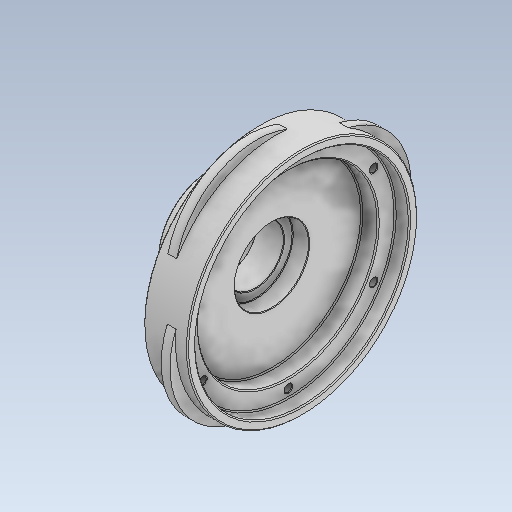
# Autodesk Inventor part: Peça21
Saved by Autodesk Inventor 2021 (Build 250183000, 183)
## iProperties
Category: 41
Created: 2021-07-19
Part Number: Peça21
Material: Genérico
Document SubType Name: Modeling
Designer: Giovanni
Density: 1 g/cm^3
Appearance: Padrão
User Status: 1:6
Author: Giovanni
Keywords: 27
Autodesk Inventor part; units mm, degrees
ref_plane "YZ Plane" through (0, 0, 0) normal (1, 0, 0) x (0, 1, 0)
sketch "Esboço1" plane through (0, 0, 0) normal (0, 0, 1) x (1, 0, 0)
  line L0 (0, 0) -> (100, 0)
  line L1 (0, 0) -> (0, 47.5)
  line L2 (0, 47.5) -> (35, 47.5)
  line L3 (35, 47.5) -> (35, 90)
  line L4 (35, 90) -> (45, 90)
  line L5 (45, 90) -> (45, 105)
  line L6 (45, 105) -> (85, 105)
  line L7 (85, 105) -> (85, 0)
  line L8 (85, 0) -> (0, 0)
  point P0 (85, 0)
  dimension "d0" = 100
  dimension "d1" = 95
  dimension "d2" = 180
  dimension "d3" = 210
  dimension "d4" = 35
  dimension "d5" = 10
  dimension "d6" = 40
  constraints: 18 end point, 6 perpendicular, 1 horizontal
  measures "d0" distance of L0.start L0.end
  measures "d1" diameter of L2 L0
  measures "d2" diameter of L4 L0
  measures "d3" diameter of L6 L0
  measures "d4" distance of L1.end L2.end
  measures "d5" distance of L3.end L4.end
  measures "d6" distance of L5.end L6.end
revolve "Revolução1" add sketch "Esboço1" angle 360 about axis through (0, 0, 0) along (1, 0, 0)
sketch "Esboço2" plane through (0, 0, 0) normal (0, 0, 1) x (1, 0, 0)
  line L0 (0, 0) -> (85, 0)
  line L1 (85, -105) -> (85, 105) projected
  line L2 (85, 0) -> (85, 97.5)
  line L3 (85, 97.5) -> (72, 97.5)
  line L4 (72, 97.5) -> (72, 82)
  line L5 (72, 82) -> (57, 82)
  line L6 (57, 82) -> (57, 0)
  line L7 (85, 0) -> (57, 0)
  dimension "d8" = 195
  dimension "d9" = 164
  dimension "d10" = 13
  dimension "d11" = 28
  constraints: 14 end point, 2 point on line, 1 collinear, 1 horizontal, 1 midpoint, 1 parallel, 1 perpendicular
  measures "d8" diameter of L3 L0
  measures "d9" diameter of L5 L0
  measures "d10" distance of L2.end L3.end
  measures "d11" distance from line of L6 L2.end
revolve "Revolução2" cut sketch "Esboço2" angle 360 about axis through (0, 0, 0) along (1, 0, 0)
sketch "Esboço3" plane through (0, 0, 0) normal (0, 0, 1) x (1, 0, 0)
  line L0 (0, 0) -> (57, 0)
  line L1 (57, 82) -> (57, -82) projected
  line L2 (0, 0) -> (0, 34)
  line L3 (0, -47.5) -> (0, 47.5) projected
  line L4 (0, 34) -> (17, 34)
  line L5 (17, 34) -> (17, 26)
  line L6 (17, 26) -> (42, 26)
  line L7 (42, 26) -> (42, 34)
  line L8 (42, 34) -> (57, 34)
  line L9 (57, 34) -> (57, 0)
  dimension "d13" = 68
  dimension "d14" = 52
  dimension "d15" = 17
  dimension "d16" = 15
  constraints: 16 end point, 4 point on line, 1 collinear, 1 midpoint
  measures "d13" diameter of L4 L0
  measures "d14" diameter of L6 L0
  measures "d15" distance of L2.end L4.end
  measures "d16" distance of L7.end L8.end
revolve "Revolução3" cut sketch "Esboço3" angle 360 about axis through (0, 0, 0) along (1, 0, 0)
ref_plane "Plano de trabalho1" through (74, 0, 0) normal (1, 0, 0) x (0, 0, -1)
sketch "Esboço4" plane through (74, 0, 0) normal (1, 0, 0) x (0, 0, -1)
  arc A0 (104.5056, -10.1775) -> (52.5086, 90.9277) centre (35, 18) ccw
  circle A1 centre (0, 0) radius 105 projected
  dimension "d19" = 150
  dimension "d20" = 18
  dimension "d21" = 35
  constraints: 4 point on circle, 1 centre point
  measures "d19" diameter of A0
  measures "d20" vertical distance of A0.centre point (0, 0)
  measures "d21" horizontal distance of point (0, 0) A0.centre
extrude "Extrusão1" add sketch "Esboço4" against normal blind 8 contours A1 A0
pattern_circular "Padrão circular1" count 2 over 360 about axis through (65, 0, 0) along (1, 0, 0) of "Extrusão1"
ref_plane "Plano de trabalho2" through (61, 0, 0) normal (1, 0, 0) x (0, 0, -1)
sketch "Esboço5" plane through (61, 0, 0) normal (1, 0, 0) x (0, 0, -1)
  arc A0 (10.1775, 104.5056) -> (-90.9277, 52.5086) centre (-18, 35) ccw
  circle A1 centre (0, 0) radius 105 projected
  dimension "d28" = 18
  dimension "d29" = 35
  dimension "d30" = 150
  constraints: 4 point on circle, 1 centre point
  measures "d28" horizontal distance of point (0, 0) A0.centre
  measures "d29" vertical distance of point (0, 0) A0.centre
  measures "d30" diameter of A0
extrude "Extrusão2" add sketch "Esboço5" against normal blind 8 contours A1 A0
pattern_circular "Padrão circular2" count 2 over 360 about axis through (-10, 0, 0) along (1, 0, 0) of "Extrusão2"
sketch "Esboço6" plane through (0, 0, 0) normal (-1, 0, 0) x (0, 0, 1)
  circle A0 centre (0, 0) radius 34 projected
  point P0 (0, 40)
  dimension "d36" = 40
  constraints: 1 vertical alignment
  measures "d36" distance of A0.centre point (0, 40)
hole "Furo1" at (0, 40, 0) direction (1, 0, 0) diameter 4.917 depth 18 tip angle 118 thread size "M6x1" class "6H" standard "ANSI Metric M Profile"
chamfer "Chanfro1" distance 0.5 angle 45 1 edges at (0, 40, -2.4585)
pattern_circular "Padrão circular3" count 4 over 360 about axis through (-10, 0, 0) along (1, 0, 0) of "Furo1", "Chanfro1"
sketch "Esboço7" plane through (72, 0, 0) normal (1, 0, 0) x (0, 0, -1)
  circle A0 centre (0, 0) radius 82 projected
  point P0 (0, 90)
  dimension "d50" = 90
  constraints: 1 vertical alignment
  measures "d50" distance of A0.centre point (0, 90)
hole "Furo2" at (72, 90, 0) direction (-1, 0, 0) diameter 6.917 depth 20 tip angle 118 thread size "M8x1" class "6H" standard "ANSI Metric M Profile"
chamfer "Chanfro2" distance 0.5 angle 45 1 edges at (72, 90, 3.4585)
pattern_circular "Padrão circular4" count 6 over 360 about axis through (-10, 0, 0) along (1, 0, 0) of "Furo2", "Chanfro2"
chamfer "Chanfro3" distance 0.5 angle 45 5 edges at (57, -34, 0) (42, -34, 0) (42, -26, 0) (17, -26, 0) (17, -34, 0)
chamfer "Chanfro4" distance 0.5 angle 45 1 edges at (0, -34, 0)
chamfer "Chanfro5" distance 1 angle 45 10 edges at (0, -47.5, 0) (35, -47.5, 0) (35, -90, 0) (45, -90, 0) (45, -105, 0) (85, -105, 0) (85, -97.5, 0) (72, -97.5, 0) (72, -82, 0) (57, -82, 0)
